Links  big screw 3_v7 (Autodesk Fusion 360 design; units mm, degrees)
Autodesk Fusion 360 part; units mm, degrees
note: some values were not read from the file. Chosen so that the rebuilt part matches the saved one: which face or edge a step refers to. Set by a fixed rule: which sketch regions a step uses.
sketch "passive link sketch" plane through (0, 0, 0) normal (0, 0, 1) x (1, 0, 0)
  line L0 (-16.4533, 8) -> (-16.4533, -8) construction
  line L1 (16.4533, -8) -> (16.4533, 8) construction
  line L2 (16.4533, 8) -> (-16.4533, -8) construction
  line L3 (-16.4533, 8) -> (16.4533, -8) construction
  circle A0 centre (12.5, 0) radius 4.5
  circle A1 centre (12.5, 0) radius 2.975
  circle A2 centre (12.5, 0) radius 8
  line L4 (0, 8) -> (0, -15) construction
  line L5 (12.5, 8) -> (0, 8)
  line L6 (0, -8) -> (12.5, -8)
  line L7 (12.5, -8) -> (12.5, 8)
  line L8 (12.5, 8) -> (-12.5, -8) construction
  line L9 (-12.5, 8) -> (12.5, -8) construction
  line L10 (16.4533, 8) -> (0, 8) construction
  line L11 (-12.5, 8) -> (-16.4533, 8) construction
  line L12 (-16.4533, -8) -> (-12.5, -8) construction
  line L13 (0, -8) -> (16.4533, -8) construction
  line L14 (0, -8) -> (-16.4533, -8) construction
  line L15 (-12.5, -8) -> (-12.5, 8)
  line L16 (-16.4533, 8) -> (0, 8) construction
  circle A3 centre (-12.5, 0) radius 8
  circle A4 centre (-12.5, 0) radius 2.975
  circle A5 centre (-12.5, 0) radius 4.5
  line L17 (0, -8) -> (-12.5, -8)
  line L18 (-12.5, 8) -> (0, 8)
  dimension "d2" = 16
  dimension "d3" = 9
  dimension "d4" = 5.95
  dimension "d5" = 16
  dimension "d6" = 12.5
  dimension "d7" = 25
  constraint horizontal L10
  constraint perpendicular L0 L10
  constraint parallel L10 L12
  constraint parallel L0 L1
  constraint coincident L2 origin
  constraint coincident L3 origin
  constraint concentric A0 A1
  constraint concentric A0 A2
  constraint perpendicular L4 L12
  constraint horizontal origin A0.centre
  constraint horizontal L5
  constraint parallel L5 L6
  constraint coincident A2 L5.start
  constraint coincident L8 origin
  constraint coincident L9 origin
  constraint collinear L10 L11
  constraint coincident L4 L6.start
  constraint collinear L12 L13
  constraint symmetric L1.end L4 L0.start
  constraint symmetric L1.start L4 L0.end
  constraint symmetric A0 L4 A5
  constraint symmetric A1 L4 A4
  constraint symmetric A2 L4 A3
  constraint symmetric L4 L5.start L9.start
  constraint symmetric L4 L6.end L8.end
  constraint symmetric L4 L5.end L10.end
  constraint symmetric L4 L6.start L13.start
  constraint perpendicular L15 L18
  constraint coincident L4 origin
  measures "d2" distance of L0.start L0.end
  measures "d3" diameter of A0
  measures "d4" diameter of A1
  measures "d5" diameter of A2
  measures "d6" distance of origin A0.centre
  measures "d7" distance of L8.end L6.end
extrude "base" add sketch "passive link sketch" along normal mid plane 4 contours A0 A1 L7 | A0 A2 L7 | A2 L5 L6 A3 L17 L18 | L15 A3 A5 | L15 A4 A5 picked at (11.6865, -3.8972) picked at (12.1026, -6.8035) picked at (-12.1205, 6.8062) picked at (-11.7228, 3.9055) makes body 1
extrude "l  big cyl" add sketch "passive link sketch" along normal blind 5 and the other way blind 6 separate body contours L15 A3 A5 | L15 A3 A5 | L15 A4 A5 | L15 A4 A5 makes body 2
fillet "Fillet13" radius 3 1 edges at (-19.9586, 2.8929, -6) on bodies 2
fillet "Fillet9" radius 0.3 1 edges at (-19.9586, -2.8929, 5) on bodies 2
extrude "Extrude8" add sketch "passive link sketch" along normal blind 5 and the other way blind 7 separate body contours L15 A4 A5 | L15 A4 A5 makes body 3
sketch "Square nut hole" plane through (0, 0, 5) normal (0, 0, 1) x (1, 0, 0)
  circle A0 centre (-12.5, 0) radius 2.975
  line L0 (-18, 5.5) -> (-7, 5.5)
  line L1 (-7, 5.5) -> (-7, -5.5)
  line L2 (-7, -5.5) -> (-18, -5.5)
  line L3 (-18, -5.5) -> (-18, 5.5)
  line L4 (-18, 5.5) -> (-7, -5.5) construction
  line L5 (-7, 5.5) -> (-18, -5.5) construction
  circle A1 centre (-12.5, 0) radius 7.7
  point P0 (-12.5, 0)
  dimension "d148" = 11
  dimension "d149" = 11
  constraint horizontal L0
  constraint perpendicular L0 L1
  constraint parallel L0 L2
  constraint parallel L1 L3
  constraint coincident L4 P0
  constraint coincident L5 P0
  constraint coincident P0 A0.centre
  measures "d148" distance of L1.end L2.end
  measures "d149" distance of L0.end L1.end
extrude "Extrude17" cut sketch "Square nut hole" against normal blind 4 contours L0 L3 A1 | L0 L1 L2 L3 A1 | L0 L1 A1 | L2 L3 A1 | L1 L2 A1 bodies 2 3
fillet "Fillet14" radius 0.3 1 edges at (-16.6955, 1.6273, -7) on bodies 3
mirror "Mirror1" about plane through (0, 0, 0) normal (1, 0, 0) of bodies 2 3 makes body 4 at (4.5398, 0.7965, -0.4333) makes body 5 at (8.0224, -0.4481, -4.1333)
mirror "Mirror2" about plane through (0, 0, 0) normal (0, 0, 1) of bodies 4 5 makes body 6 at (4.5398, 0.7965, 0.4333) makes body 7 at (8.0224, -0.4481, 4.1333)
delete_body "RemoveBody1" bodies 4
delete_body "RemoveBody2" bodies 5
sketch "motorLinkSketch" plane through (0, 0, 0) normal (0, 0, 1) x (1, 0, 0) in component "MotorLinkComponent"
  line L0 (0, 8) -> (0, -15.0002) construction
  line L1 (0, -8) -> (16.4996, -8) construction
  circle A0 centre (-12.5, 0) radius 8
  line L2 (0, -8) -> (-16.4996, -8) construction
  circle A1 centre (-12.5, 0) radius 2.975
  line L3 (-16.4996, -8) -> (-12.5, -8) construction
  line L4 (-12.5, 8) -> (0, 8)
  circle A2 centre (12.5, 0) radius 2.975
  line L5 (16.4996, 8) -> (0, 8) construction
  circle A3 centre (-12.5, 0) radius 2.975
  line L6 (0, -8) -> (-12.5, -8)
  line L7 (-16.4996, 8) -> (0, 8) construction
  line L8 (-12.5, -8) -> (-12.5, 8)
  circle A4 centre (12.5, 0) radius 2.975
  line L9 (-12.5, 8) -> (12.5, -8) construction
  line L10 (-16.4996, 8) -> (16.4996, -8) construction
  line L11 (12.5, 8) -> (0, 8)
  line L12 (-16.4996, 8) -> (-16.4996, -8) construction
  line L13 (-12.5, 8) -> (-16.4996, 8) construction
  line L14 (12.5, 8) -> (-12.5, -8) construction
  line L15 (16.4996, 8) -> (-16.4996, -8) construction
  line L16 (12.5, -8) -> (12.5, 8)
  line L17 (16.4996, -8) -> (16.4996, 8) construction
  circle A5 centre (12.5, 0) radius 8
  line L18 (0, -8) -> (12.5, -8)
  line L19 (14.65, 2.0562) -> (14.65, -2.0562)
  dimension "d157" = 16
  dimension "d158" = 5.95
  dimension "d159" = 5.95
  dimension "d160" = 16
  dimension "d161" = 12.5
  dimension "d162" = 25
  dimension "d163" = 2.15
  constraint horizontal L5
  constraint perpendicular L5 L12
  constraint parallel L3 L5
  constraint parallel L12 L17
  constraint coincident origin L15
  constraint coincident origin L10
  constraint concentric A2 A4
  constraint concentric A4 A5
  constraint perpendicular L0 L3
  constraint horizontal A2.centre origin
  constraint horizontal L11
  constraint parallel L11 L18
  constraint coincident L11.start A5
  constraint coincident origin L14
  constraint coincident origin L9
  constraint collinear L5 L13
  constraint coincident L1.start L0
  constraint collinear L1 L3
  constraint symmetric L5.start L7.start L0
  constraint symmetric L1.end L2.end L0
  constraint symmetric L0 A3 A4
  constraint symmetric L0 A1 A2
  constraint symmetric L0 A0 A5
  constraint symmetric L11.start L4.start L0
  constraint symmetric L3.end L9.end L0
  constraint symmetric L4.end L5.end L0
  constraint symmetric L1.start L2.start L0
  constraint perpendicular L4 L8
  constraint coincident origin L0
  constraint coincident A2 L19.start
  constraint coincident A2 L19.end
  constraint vertical L19
  measures "d157" distance of L2.end L7.start
  measures "d158" diameter of A4
  measures "d159" diameter of A2
  measures "d160" diameter of A5
  measures "d161" distance of A2.centre origin
  measures "d162" distance of L3.end L9.end
  measures "d163" distance of A2.centre L19
extrude "Extrude10" [suppressed] in component "MotorLinkComponent"
extrude "Extrude11" [suppressed] in component "MotorLinkComponent"
fillet "Fillet4" [suppressed] in component "MotorLinkComponent"
sketch "Sketch3" plane through (0, 0, 5) normal (0, 0, 1) x (-1, 0, 0) in component "MotorLinkComponent"
  circle A0 centre (12.5, 0) radius 2.975
  circle A1 centre (12.5, 0) radius 7.7
  line L0 (18, -5.5) -> (7, -5.5)
  line L1 (7, -5.5) -> (7, 5.5)
  line L2 (7, 5.5) -> (18, 5.5)
  line L3 (18, 5.5) -> (18, -5.5)
  line L4 (18, -5.5) -> (7, 5.5) construction
  line L5 (7, -5.5) -> (18, 5.5) construction
  point P0 (12.5, 0)
  dimension "d192" = 11
  dimension "d193" = 11
  constraint horizontal L0
  constraint perpendicular L0 L1
  constraint parallel L0 L2
  constraint parallel L1 L3
  constraint coincident L4 P0
  constraint coincident L5 P0
  constraint coincident P0 A0.centre
  measures "d192" distance of L1.end L2.end
  measures "d193" distance of L0.end L1.end
extrude "Extrude12" [suppressed] in component "MotorLinkComponent"
extrude "Extrude9" [suppressed] in component "MotorLinkComponent"
extrude "Extrude8'" [suppressed] in component "MotorLinkComponent"
extrude "Extrude18" [suppressed]
extrude "Extrude19" [suppressed]
sketch "spacer" plane through (0, 0, 0) normal (0, 0, 1) x (1, 0, 0)
  circle A0 centre (-61, 0) radius 4
  circle A1 centre (-61, 0) radius 1
  dimension "d123" = 8
  dimension "d126" = 2
  constraint concentric A0 A1
  measures "d123" diameter of A0
  measures "d126" diameter of A1
extrude "Extrude16" [suppressed]
component "MotorLinkComponent" placed x (1, 0, 0) y (0, 1, 0) z (0, 0, 1) at (40, 0, 0)
equation "d2 = BigBarrelDiam"
equation "d3 = restShoulderDiam"
equation "d4 = smallerHoleDiam"
equation "d5 = BigBarrelDiam"
equation "d8 = rect / 2"
equation "d16 = bigBarrelNutSideHeight"
equation "d22 = bigBarrelNutSideHeight"
equation "d24 = bigBarrelScrewSideHeight"
equation "d25 = 0.0 °"
equation "d52 = bigBarrelScrewSideHeight - 1 mm"
equation "d53 = 0.0 °"
equation "rect = 4 mm"
equation "nipDiameterXXX = 5.95 mm"
equation "BigBarrelDiam = 16 mm"
equation "smallerHoleDiam = 5.95 mm"
equation "motorShaftDiameter = 5.2 mm"
equation "shaftNipDiam = 5.9 mm"
equation "rectLen = 25 mm"
equation "d134 = -nutDepth"
equation "d157 = BigBarrelDiam"
equation "d158 = smallerHoleDiam"
equation "d159 = nipDiameterXXX"
equation "d160 = BigBarrelDiam"
equation "d161 = rectLen / 2"
equation "d162 = rectLen"
equation "d164 = rect / 2 + shaftNipDiam"
equation "d166 = rect / 2"
equation "d167 = 0.0 °"
equation "d168 = rect / 2 + shaftNipDiam"
equation "d170 = rect / 2"
equation "d171 = 0.0 °"
equation "d172 = rect / 2 + 8 mm"
equation "d175 = 0.0 °"
equation "d176 = rect / 2 + 8 mm"
equation "d179 = 0.0 °"
equation "d180 = rect / 2"
equation "d187 = 0.0 °"
equation "restShoulderDiam = 9 mm"
equation "bigBarrelNutSideHeight = 5 mm"
equation "bigBarrelScrewSideHeight = 7 mm"
equation "restShoulderHeight = 33 mm"
equation "nutDepth = 4 mm"
named bodies: "spacer", "big barrel", "screwHole", "big barrel (1)", "screwHole (1)", "big barrel (1) (1)", "screwHole (1) (1)", "big barrel for shaft", "cuboid", "big barrel with screw"
